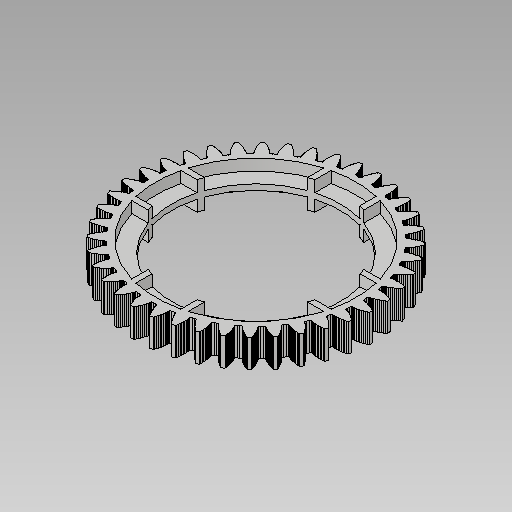
# Autodesk Inventor part: gear40
Saved by Autodesk Inventor 2020 (Build 240168000, 168)
## iProperties
Created: 2018-12-28
Part Number: gear40
Material: Generic
Document SubType Name: Modeling
Designer: Varga Daniel
Density: 1 g/cm^3
Appearance: Default
Sending System: SolidWorks 2018
Last Author: david
Last Saved: 2018-12-28
Author: Varga Daniel
Autodesk Inventor part; units mm, degrees
(part 1 of 3)
ref_plane "YZ Plane" through (0, 0, 0) normal (1, 0, 0) x (0, 1, 0)
ref_plane "XZ Plane" through (0, 0, 0) normal (0, 1, 0) x (-1, 0, 0)
ref_plane "XY Plane" through (0, 0, 0) normal (0, 0, 1) x (1, 0, 0)
sketch "Gear 40 tooth shape" plane through (0, 0, 0) normal (0, 0, 1) x (1, 0, 0)
  line L0 (2.4506, 21.4015) -> (2.3942, 21.6857)
  line L1 (2.3942, 21.6857) -> (2.3331, 21.6926)
  line L2 (2.3331, 21.6926) -> (2.2721, 21.7014)
  line L3 (2.2721, 21.7014) -> (2.1501, 21.7236)
  line L4 (2.1501, 21.7236) -> (2.0283, 21.7505)
  line L5 (2.0283, 21.7505) -> (1.9066, 21.7815)
  line L6 (1.9066, 21.7815) -> (1.6637, 21.8541)
  line L7 (1.6637, 21.8541) -> (1.4215, 21.9391)
  line L8 (1.4215, 21.9391) -> (1.18, 22.0351)
  line L9 (1.18, 22.0351) -> (0.9394, 22.1414)
  line L10 (0.9394, 22.1414) -> (0.6996, 22.2573)
  line L11 (0.6996, 22.2573) -> (0.461, 22.3824)
  line L12 (0.461, 22.3824) -> (0.2234, 22.5162)
  line L13 (0.2234, 22.5162) -> (0.046, 22.6222)
  line L14 (0.046, 22.6222) -> (0.0882, 23.1579)
  line L15 (0.0882, 23.1579) -> (0.2799, 23.2348)
  line L16 (0.2799, 23.2348) -> (0.5355, 23.3299)
  line L17 (0.5355, 23.3299) -> (0.7908, 23.4161)
  line L18 (0.7908, 23.4161) -> (1.0457, 23.4931)
  line L19 (1.0457, 23.4931) -> (1.3001, 23.5604)
  line L20 (1.3001, 23.5604) -> (1.5536, 23.6175)
  line L21 (1.5536, 23.6175) -> (1.8061, 23.6635)
  line L22 (1.8061, 23.6635) -> (2.0574, 23.6972)
  line L23 (2.0574, 23.6972) -> (2.1824, 23.7088)
  line L24 (2.1824, 23.7088) -> (2.3069, 23.7163)
  line L25 (2.3069, 23.7163) -> (2.4309, 23.7191)
  line L26 (2.4309, 23.7191) -> (2.4925, 23.7183)
  line L27 (2.4925, 23.7183) -> (2.554, 23.7155)
  line L28 (2.554, 23.7155) -> (2.6542, 23.9874)
  line L29 (2.6542, 23.9874) -> (2.7094, 24.3363)
  line L30 (2.7094, 24.3363) -> (2.6981, 24.6258)
  line L31 (2.6981, 24.6258) -> (2.6389, 24.6422)
  line L32 (2.6389, 24.6422) -> (2.58, 24.6605)
  line L33 (2.58, 24.6605) -> (2.463, 24.7014)
  line L34 (2.463, 24.7014) -> (2.3469, 24.7471)
  line L35 (2.3469, 24.7471) -> (2.2315, 24.7967)
  line L36 (2.2315, 24.7967) -> (2.003, 24.9064)
  line L37 (2.003, 24.9064) -> (1.777, 25.0282)
  line L38 (1.777, 25.0282) -> (1.5536, 25.1608)
  line L39 (1.5536, 25.1608) -> (1.3325, 25.3035)
  line L40 (1.3325, 25.3035) -> (1.1139, 25.4555)
  line L41 (1.1139, 25.4555) -> (0.8977, 25.6163)
  line L42 (0.8977, 25.6163) -> (0.684, 25.7857)
  line L43 (0.684, 25.7857) -> (0.5254, 25.9181)
  line L44 (0.5254, 25.9181) -> (0.6508, 26.4406)
  line L45 (0.6508, 26.4406) -> (0.8522, 26.4866)
  line L46 (0.8522, 26.4866) -> (1.1195, 26.5405)
  line L47 (1.1195, 26.5405) -> (1.3852, 26.5857)
  line L48 (1.3852, 26.5857) -> (1.649, 26.6219)
  line L49 (1.649, 26.6219) -> (1.9107, 26.6486)
  line L50 (1.9107, 26.6486) -> (2.1701, 26.6653)
  line L51 (2.1701, 26.6653) -> (2.4267, 26.6713)
  line L52 (2.4267, 26.6713) -> (2.6801, 26.6652)
  line L53 (2.6801, 26.6652) -> (2.8054, 26.6571)
  line L54 (2.8054, 26.6571) -> (2.9296, 26.6451)
  line L55 (2.9296, 26.6451) -> (3.0524, 26.6284)
  line L56 (3.0524, 26.6284) -> (3.1132, 26.618)
  line L57 (3.1132, 26.618) -> (3.1734, 26.6057)
  line L58 (3.1734, 26.6057) -> (3.315, 26.8585)
  line L59 (3.315, 26.8585) -> (3.4241, 27.1944)
  line L60 (3.4241, 27.1944) -> (3.4583, 27.4822)
  line L61 (3.4583, 27.4822) -> (3.4023, 27.5076)
  line L62 (3.4023, 27.5076) -> (3.3469, 27.5349)
  line L63 (3.3469, 27.5349) -> (3.2378, 27.5936)
  line L64 (3.2378, 27.5936) -> (3.1303, 27.6569)
  line L65 (3.1303, 27.6569) -> (3.0241, 27.724)
  line L66 (3.0241, 27.724) -> (2.8156, 27.868)
  line L67 (2.8156, 27.868) -> (2.6115, 28.0237)
  line L68 (2.6115, 28.0237) -> (2.4115, 28.1897)
  line L69 (2.4115, 28.1897) -> (2.2154, 28.3651)
  line L70 (2.2154, 28.3651) -> (2.0233, 28.5494)
  line L71 (2.0233, 28.5494) -> (1.8349, 28.7421)
  line L72 (1.8349, 28.7421) -> (1.6503, 28.9428)
  line L73 (1.6503, 28.9428) -> (1.5144, 29.0984)
  line L74 (1.5144, 29.0984) -> (1.72, 29.5949)
  line L75 (1.72, 29.5949) -> (1.9262, 29.6088)
  line L76 (1.9262, 29.6088) -> (2.1986, 29.6202)
  line L77 (2.1986, 29.6202) -> (2.4681, 29.6233)
  line L78 (2.4681, 29.6233) -> (2.7343, 29.6178)
  line L79 (2.7343, 29.6178) -> (2.997, 29.6032)
  line L80 (2.997, 29.6032) -> (3.2557, 29.5791)
  line L81 (3.2557, 29.5791) -> (3.5101, 29.5449)
  line L82 (3.5101, 29.5449) -> (3.7595, 29.4993)
  line L83 (3.7595, 29.4993) -> (3.882, 29.4717)
  line L84 (3.882, 29.4717) -> (4.0027, 29.4404)
  line L85 (4.0027, 29.4404) -> (4.1215, 29.4047)
  line L86 (4.1215, 29.4047) -> (4.1799, 29.3849)
  line L87 (4.1799, 29.3849) -> (4.2374, 29.3633)
  line L88 (4.2374, 29.3633) -> (4.4167, 29.5909)
  line L89 (4.4167, 29.5909) -> (4.5771, 29.9056)
  line L90 (4.5771, 29.9056) -> (4.6558, 30.1845)
  line L91 (4.6558, 30.1845) -> (4.6045, 30.2183)
  line L92 (4.6045, 30.2183) -> (4.5541, 30.2539)
  line L93 (4.5541, 30.2539) -> (4.4555, 30.329)
  line L94 (4.4555, 30.329) -> (4.3592, 30.4083)
  line L95 (4.3592, 30.4083) -> (4.2649, 30.4912)
  line L96 (4.2649, 30.4912) -> (4.0814, 30.6661)
  line L97 (4.0814, 30.6661) -> (3.9042, 30.8518)
  line L98 (3.9042, 30.8518) -> (3.7326, 31.047)
  line L99 (3.7326, 31.047) -> (3.5664, 31.2509)
  line L100 (3.5664, 31.2509) -> (3.4055, 31.4631)
  line L101 (3.4055, 31.4631) -> (3.2496, 31.6829)
  line L102 (3.2496, 31.6829) -> (3.0987, 31.91)
  line L103 (3.0987, 31.91) -> (2.9888, 32.0849)
  line L104 (2.9888, 32.0849) -> (3.2695, 32.5431)
  line L105 (3.2695, 32.5431) -> (3.4753, 32.5246)
  line L106 (3.4753, 32.5246) -> (3.7462, 32.4932)
  line L107 (3.7462, 32.4932) -> (4.0128, 32.4541)
  line L108 (4.0128, 32.4541) -> (4.2749, 32.407)
  line L109 (4.2749, 32.407) -> (4.532, 32.3515)
  line L110 (4.532, 32.3515) -> (4.7839, 32.2873)
  line L111 (4.7839, 32.2873) -> (5.0298, 32.2137)
  line L112 (5.0298, 32.2137) -> (5.2689, 32.1296)
  line L113 (5.2689, 32.1296) -> (5.3856, 32.0832)
  line L114 (5.3856, 32.0832) -> (5.5, 32.0334)
  line L115 (5.5, 32.0334) -> (5.6116, 31.9796)
  line L116 (5.6116, 31.9796) -> (5.6662, 31.9509)
  line L117 (5.6662, 31.9509) -> (5.7197, 31.9205)
  line L118 (5.7197, 31.9205) -> (5.9324, 32.1173)
  line L119 (5.9324, 32.1173) -> (6.14, 32.403)
  line L120 (6.14, 32.403) -> (6.2614, 32.6661)
  line L121 (6.2614, 32.6661) -> (6.216, 32.7076)
  line L122 (6.216, 32.7076) -> (6.1718, 32.7506)
  line L123 (6.1718, 32.7506) -> (6.0862, 32.8402)
  line L124 (6.0862, 32.8402) -> (6.0035, 32.9336)
  line L125 (6.0035, 32.9336) -> (5.9233, 33.0302)
  line L126 (5.9233, 33.0302) -> (5.7694, 33.2317)
  line L127 (5.7694, 33.2317) -> (5.6234, 33.4428)
  line L128 (5.6234, 33.4428) -> (5.4845, 33.6624)
  line L129 (5.4845, 33.6624) -> (5.3523, 33.8899)
  line L130 (5.3523, 33.8899) -> (5.2265, 34.1246)
  line L131 (5.2265, 34.1246) -> (5.1069, 34.3661)
  line L132 (5.1069, 34.3661) -> (4.9934, 34.614)
  line L133 (4.9934, 34.614) -> (4.9122, 34.804)
  line L134 (4.9122, 34.804) -> (5.2611, 35.2126)
  line L135 (5.2611, 35.2126) -> (5.4615, 35.1621)
  line L136 (5.4615, 35.1621) -> (5.7241, 35.0888)
  line L137 (5.7241, 35.0888) -> (5.9813, 35.0084)
  line L138 (5.9813, 35.0084) -> (6.2328, 34.9209)
  line L139 (6.2328, 34.9209) -> (6.4781, 34.8259)
  line L140 (6.4781, 34.8259) -> (6.7168, 34.723)
  line L141 (6.7168, 34.723) -> (6.9482, 34.6118)
  line L142 (6.9482, 34.6118) -> (7.1712, 34.4914)
  line L143 (7.1712, 34.4914) -> (7.2792, 34.4273)
  line L144 (7.2792, 34.4273) -> (7.3844, 34.3602)
  line L145 (7.3844, 34.3602) -> (7.4863, 34.2896)
  line L146 (7.4863, 34.2896) -> (7.5357, 34.2527)
  line L147 (7.5357, 34.2527) -> (7.5837, 34.2144)
  line L148 (7.5837, 34.2144) -> (7.8246, 34.3754)
  line L149 (7.8246, 34.3754) -> (8.0744, 34.6252)
  line L150 (8.0744, 34.6252) -> (8.2354, 34.8661)
  line L151 (8.2354, 34.8661) -> (8.1971, 34.9141)
  line L152 (8.1971, 34.9141) -> (8.1602, 34.9635)
  line L153 (8.1602, 34.9635) -> (8.0896, 35.0654)
  line L154 (8.0896, 35.0654) -> (8.0225, 35.1706)
  line L155 (8.0225, 35.1706) -> (7.9584, 35.2786)
  line L156 (7.9584, 35.2786) -> (7.838, 35.5016)
  line L157 (7.838, 35.5016) -> (7.7268, 35.733)
  line L158 (7.7268, 35.733) -> (7.6239, 35.9717)
  line L159 (7.6239, 35.9717) -> (7.5289, 36.217)
  line L160 (7.5289, 36.217) -> (7.4414, 36.4685)
  line L161 (7.4414, 36.4685) -> (7.361, 36.7257)
  line L162 (7.361, 36.7257) -> (7.2877, 36.9883)
  line L163 (7.2877, 36.9883) -> (7.2372, 37.1887)
  line L164 (7.2372, 37.1887) -> (7.6459, 37.5377)
  line L165 (7.6459, 37.5377) -> (7.8358, 37.4565)
  line L166 (7.8358, 37.4565) -> (8.0837, 37.343)
  line L167 (8.0837, 37.343) -> (8.3252, 37.2234)
  line L168 (8.3252, 37.2234) -> (8.5599, 37.0975)
  line L169 (8.5599, 37.0975) -> (8.7874, 36.9653)
  line L170 (8.7874, 36.9653) -> (9.007, 36.8264)
  line L171 (9.007, 36.8264) -> (9.2181, 36.6804)
  line L172 (9.2181, 36.6804) -> (9.4196, 36.5266)
  line L173 (9.4196, 36.5266) -> (9.5162, 36.4464)
  line L174 (9.5162, 36.4464) -> (9.6096, 36.3636)
  line L175 (9.6096, 36.3636) -> (9.6992, 36.278)
  line L176 (9.6992, 36.278) -> (9.7422, 36.2338)
  line L177 (9.7422, 36.2338) -> (9.7837, 36.1884)
  line L178 (9.7837, 36.1884) -> (10.0468, 36.3098)
  line L179 (10.0468, 36.3098) -> (10.3326, 36.5174)
  line L180 (10.3326, 36.5174) -> (10.5293, 36.7301)
  line L181 (10.5293, 36.7301) -> (10.499, 36.7836)
  line L182 (10.499, 36.7836) -> (10.4702, 36.8382)
  line L183 (10.4702, 36.8382) -> (10.4164, 36.9499)
  line L184 (10.4164, 36.9499) -> (10.3666, 37.0642)
  line L185 (10.3666, 37.0642) -> (10.3202, 37.1809)
  line L186 (10.3202, 37.1809) -> (10.2362, 37.4201)
  line L187 (10.2362, 37.4201) -> (10.1625, 37.666)
  line L188 (10.1625, 37.666) -> (10.0983, 37.9178)
  line L189 (10.0983, 37.9178) -> (10.0428, 38.175)
  line L190 (10.0428, 38.175) -> (9.9957, 38.437)
  line L191 (9.9957, 38.437) -> (9.9566, 38.7037)
  line L192 (9.9566, 38.7037) -> (9.9252, 38.9745)
  line L193 (9.9252, 38.9745) -> (9.9067, 39.1803)
  line L194 (9.9067, 39.1803) -> (10.3649, 39.4611)
  line L195 (10.3649, 39.4611) -> (10.5398, 39.3511)
  line L196 (10.5398, 39.3511) -> (10.7669, 39.2002)
  line L197 (10.7669, 39.2002) -> (10.9868, 39.0443)
  line L198 (10.9868, 39.0443) -> (11.1989, 38.8834)
  line L199 (11.1989, 38.8834) -> (11.4028, 38.7172)
  line L200 (11.4028, 38.7172) -> (11.5981, 38.5456)
  line L201 (11.5981, 38.5456) -> (11.7837, 38.3684)
  line L202 (11.7837, 38.3684) -> (11.9586, 38.1849)
  line L203 (11.9586, 38.1849) -> (12.0415, 38.0906)
  line L204 (12.0415, 38.0906) -> (12.1208, 37.9943)
  line L205 (12.1208, 37.9943) -> (12.1959, 37.8957)
  line L206 (12.1959, 37.8957) -> (12.2315, 37.8453)
  line L207 (12.2315, 37.8453) -> (12.2654, 37.794)
  line L208 (12.2654, 37.794) -> (12.5442, 37.8727)
  line L209 (12.5442, 37.8727) -> (12.8589, 38.0331)
  line L210 (12.8589, 38.0331) -> (13.0865, 38.2124)
  line L211 (13.0865, 38.2124) -> (13.0649, 38.27)
  line L212 (13.0649, 38.27) -> (13.0451, 38.3284)
  line L213 (13.0451, 38.3284) -> (13.0095, 38.4471)
  line L214 (13.0095, 38.4471) -> (12.9781, 38.5678)
  line L215 (12.9781, 38.5678) -> (12.9505, 38.6903)
  line L216 (12.9505, 38.6903) -> (12.9049, 38.9397)
  line L217 (12.9049, 38.9397) -> (12.8707, 39.1941)
  line L218 (12.8707, 39.1941) -> (12.8466, 39.4528)
  line L219 (12.8466, 39.4528) -> (12.8321, 39.7155)
  line L220 (12.8321, 39.7155) -> (12.8265, 39.9817)
  line L221 (12.8265, 39.9817) -> (12.8296, 40.2512)
  line L222 (12.8296, 40.2512) -> (12.841, 40.5236)
  line L223 (12.841, 40.5236) -> (12.8549, 40.7298)
  line L224 (12.8549, 40.7298) -> (13.3514, 40.9354)
  line L225 (13.3514, 40.9354) -> (13.507, 40.7995)
  line L226 (13.507, 40.7995) -> (13.7077, 40.6149)
  line L227 (13.7077, 40.6149) -> (13.9004, 40.4266)
  line L228 (13.9004, 40.4266) -> (14.0847, 40.2344)
  line L229 (14.0847, 40.2344) -> (14.2601, 40.0384)
  line L230 (14.2601, 40.0384) -> (14.4261, 39.8384)
  line L231 (14.4261, 39.8384) -> (14.5818, 39.6343)
  line L232 (14.5818, 39.6343) -> (14.7259, 39.4257)
  line L233 (14.7259, 39.4257) -> (14.7929, 39.3196)
  line L234 (14.7929, 39.3196) -> (14.8562, 39.212)
  line L235 (14.8562, 39.212) -> (14.915, 39.1029)
  line L236 (14.915, 39.1029) -> (14.9422, 39.0476)
  line L237 (14.9422, 39.0476) -> (14.9676, 38.9916)
  line L238 (14.9676, 38.9916) -> (15.2554, 39.0257)
  line L239 (15.2554, 39.0257) -> (15.5913, 39.1349)
  line L240 (15.5913, 39.1349) -> (15.8442, 39.2764)
  line L241 (15.8442, 39.2764) -> (15.8318, 39.3366)
  line L242 (15.8318, 39.3366) -> (15.8214, 39.3974)
  line L243 (15.8214, 39.3974) -> (15.8047, 39.5202)
  line L244 (15.8047, 39.5202) -> (15.7927, 39.6444)
  line L245 (15.7927, 39.6444) -> (15.7846, 39.7697)
  line L246 (15.7846, 39.7697) -> (15.7786, 40.0231)
  line L247 (15.7786, 40.0231) -> (15.7845, 40.2797)
  line L248 (15.7845, 40.2797) -> (15.8012, 40.5391)
  line L249 (15.8012, 40.5391) -> (15.828, 40.8008)
  line L250 (15.828, 40.8008) -> (15.8641, 41.0646)
  line L251 (15.8641, 41.0646) -> (15.9093, 41.3303)
  line L252 (15.9093, 41.3303) -> (15.9632, 41.5976)
  line L253 (15.9632, 41.5976) -> (16.0092, 41.799)
  line L254 (16.0092, 41.799) -> (16.5317, 41.9244)
  line L255 (16.5317, 41.9244) -> (16.6641, 41.7658)
  line L256 (16.6641, 41.7658) -> (16.8335, 41.5521)
  line L257 (16.8335, 41.5521) -> (16.9944, 41.336)
  line L258 (16.9944, 41.336) -> (17.1463, 41.1173)
  line L259 (17.1463, 41.1173) -> (17.289, 40.8963)
  line L260 (17.289, 40.8963) -> (17.4216, 40.6728)
  line L261 (17.4216, 40.6728) -> (17.5434, 40.4468)
  line L262 (17.5434, 40.4468) -> (17.6531, 40.2183)
  line L263 (17.6531, 40.2183) -> (17.7028, 40.103)
  line L264 (17.7028, 40.103) -> (17.7484, 39.9869)
  line L265 (17.7484, 39.9869) -> (17.7894, 39.8699)
  line L266 (17.7894, 39.8699) -> (17.8076, 39.8109)
  line L267 (17.8076, 39.8109) -> (17.824, 39.7517)
  line L268 (17.824, 39.7517) -> (18.1135, 39.7404)
  line L269 (18.1135, 39.7404) -> (18.4624, 39.7957)
  line L270 (18.4624, 39.7957) -> (18.7343, 39.8959)
  line L271 (18.7343, 39.8959) -> (18.7315, 39.9573)
  line L272 (18.7315, 39.9573) -> (18.7307, 40.019)
  line L273 (18.7307, 40.019) -> (18.7335, 40.1429)
  line L274 (18.7335, 40.1429) -> (18.741, 40.2674)
  line L275 (18.741, 40.2674) -> (18.7526, 40.3924)
  line L276 (18.7526, 40.3924) -> (18.7863, 40.6437)
  line L277 (18.7863, 40.6437) -> (18.8323, 40.8962)
  line L278 (18.8323, 40.8962) -> (18.8894, 41.1497)
  line L279 (18.8894, 41.1497) -> (18.9568, 41.4041)
  line L280 (18.9568, 41.4041) -> (19.0338, 41.659)
  line L281 (19.0338, 41.659) -> (19.1199, 41.9143)
  line L282 (19.1199, 41.9143) -> (19.215, 42.1699)
  line L283 (19.215, 42.1699) -> (19.2919, 42.3616)
  line L284 (19.2919, 42.3616) -> (19.8276, 42.4038)
  line L285 (19.8276, 42.4038) -> (19.9336, 42.2264)
  line L286 (19.9336, 42.2264) -> (20.0674, 41.9889)
  line L287 (20.0674, 41.9889) -> (20.1925, 41.7502)
  line L288 (20.1925, 41.7502) -> (20.3084, 41.5104)
  line L289 (20.3084, 41.5104) -> (20.4147, 41.2698)
  line L290 (20.4147, 41.2698) -> (20.5108, 41.0283)
  line L291 (20.5108, 41.0283) -> (20.5957, 40.7861)
  line L292 (20.5957, 40.7861) -> (20.6683, 40.5432)
  line L293 (20.6683, 40.5432) -> (20.6993, 40.4215)
  line L294 (20.6993, 40.4215) -> (20.7262, 40.2997)
  line L295 (20.7262, 40.2997) -> (20.7484, 40.1778)
  line L296 (20.7484, 40.1778) -> (20.7572, 40.1167)
  line L297 (20.7572, 40.1167) -> (20.7641, 40.0556)
  line L298 (20.7641, 40.0556) -> (21.0483, 39.9992)
  line L299 (21.0483, 39.9992) -> (21.4015, 39.9992)
  line L300 (21.4015, 39.9992) -> (21.6857, 40.0556)
  line L301 (21.6857, 40.0556) -> (21.6926, 40.1167)
  line L302 (21.6926, 40.1167) -> (21.7014, 40.1778)
  line L303 (21.7014, 40.1778) -> (21.7236, 40.2997)
  line L304 (21.7236, 40.2997) -> (21.7505, 40.4215)
  line L305 (21.7505, 40.4215) -> (21.7815, 40.5432)
  line L306 (21.7815, 40.5432) -> (21.8541, 40.7861)
  line L307 (21.8541, 40.7861) -> (21.9391, 41.0283)
  line L308 (21.9391, 41.0283) -> (22.0351, 41.2698)
  line L309 (22.0351, 41.2698) -> (22.1414, 41.5104)
  line L310 (22.1414, 41.5104) -> (22.2573, 41.7502)
  line L311 (22.2573, 41.7502) -> (22.3824, 41.9889)
  line L312 (22.3824, 41.9889) -> (22.5162, 42.2264)
  line L313 (22.5162, 42.2264) -> (22.6222, 42.4038)
  line L314 (22.6222, 42.4038) -> (23.1579, 42.3616)
  line L315 (23.1579, 42.3616) -> (23.2348, 42.1699)
  line L316 (23.2348, 42.1699) -> (23.3299, 41.9143)
  line L317 (23.3299, 41.9143) -> (23.4161, 41.659)
  line L318 (23.4161, 41.659) -> (23.4931, 41.4041)
  line L319 (23.4931, 41.4041) -> (23.5604, 41.1497)
  line L320 (23.5604, 41.1497) -> (23.6175, 40.8962)
  line L321 (23.6175, 40.8962) -> (23.6635, 40.6437)
  line L322 (23.6635, 40.6437) -> (23.6972, 40.3924)
  line L323 (23.6972, 40.3924) -> (23.7088, 40.2674)
  line L324 (23.7088, 40.2674) -> (23.7163, 40.1429)
  line L325 (23.7163, 40.1429) -> (23.7191, 40.019)
  line L326 (23.7191, 40.019) -> (23.7183, 39.9573)
  line L327 (23.7183, 39.9573) -> (23.7155, 39.8959)
  line L328 (23.7155, 39.8959) -> (23.9874, 39.7957)
  line L329 (23.9874, 39.7957) -> (24.3363, 39.7404)
  line L330 (24.3363, 39.7404) -> (24.6258, 39.7517)
  line L331 (24.6258, 39.7517) -> (24.6422, 39.8109)
  line L332 (24.6422, 39.8109) -> (24.6605, 39.8699)
  line L333 (24.6605, 39.8699) -> (24.7014, 39.9869)
  line L334 (24.7014, 39.9869) -> (24.7471, 40.103)
  line L335 (24.7471, 40.103) -> (24.7967, 40.2183)
  line L336 (24.7967, 40.2183) -> (24.9064, 40.4468)
  line L337 (24.9064, 40.4468) -> (25.0282, 40.6728)
  line L338 (25.0282, 40.6728) -> (25.1608, 40.8963)
  line L339 (25.1608, 40.8963) -> (25.3035, 41.1173)
  line L340 (25.3035, 41.1173) -> (25.4555, 41.336)
  line L341 (25.4555, 41.336) -> (25.6163, 41.5521)
  line L342 (25.6163, 41.5521) -> (25.7857, 41.7658)
  line L343 (25.7857, 41.7658) -> (25.9181, 41.9244)
  line L344 (25.9181, 41.9244) -> (26.4406, 41.799)
  line L345 (26.4406, 41.799) -> (26.4866, 41.5976)
  line L346 (26.4866, 41.5976) -> (26.5405, 41.3303)
  line L347 (26.5405, 41.3303) -> (26.5857, 41.0646)
  line L348 (26.5857, 41.0646) -> (26.6219, 40.8008)
  line L349 (26.6219, 40.8008) -> (26.6486, 40.5391)
  line L350 (26.6486, 40.5391) -> (26.6653, 40.2797)
  line L351 (26.6653, 40.2797) -> (26.6713, 40.0231)
  line L352 (26.6713, 40.0231) -> (26.6652, 39.7697)
  line L353 (26.6652, 39.7697) -> (26.6571, 39.6444)
  line L354 (26.6571, 39.6444) -> (26.6451, 39.5202)
  line L355 (26.6451, 39.5202) -> (26.6284, 39.3974)
  line L356 (26.6284, 39.3974) -> (26.618, 39.3366)
  line L357 (26.618, 39.3366) -> (26.6057, 39.2764)
  line L358 (26.6057, 39.2764) -> (26.8585, 39.1349)
  line L359 (26.8585, 39.1349) -> (27.1944, 39.0257)
  line L360 (27.1944, 39.0257) -> (27.4822, 38.9916)
  line L361 (27.4822, 38.9916) -> (27.5076, 39.0476)
  line L362 (27.5076, 39.0476) -> (27.5349, 39.1029)
  line L363 (27.5349, 39.1029) -> (27.5936, 39.212)
  line L364 (27.5936, 39.212) -> (27.6569, 39.3196)
  line L365 (27.6569, 39.3196) -> (27.724, 39.4257)
  line L366 (27.724, 39.4257) -> (27.868, 39.6343)
  line L367 (27.868, 39.6343) -> (28.0237, 39.8384)
  line L368 (28.0237, 39.8384) -> (28.1897, 40.0384)
  line L369 (28.1897, 40.0384) -> (28.3651, 40.2344)
  line L370 (28.3651, 40.2344) -> (28.5494, 40.4266)
  line L371 (28.5494, 40.4266) -> (28.7421, 40.6149)
  line L372 (28.7421, 40.6149) -> (28.9428, 40.7995)
  line L373 (28.9428, 40.7995) -> (29.0984, 40.9354)
  line L374 (29.0984, 40.9354) -> (29.5949, 40.7298)
  line L375 (29.5949, 40.7298) -> (29.6088, 40.5236)
  line L376 (29.6088, 40.5236) -> (29.6202, 40.2512)
  line L377 (29.6202, 40.2512) -> (29.6233, 39.9817)
  line L378 (29.6233, 39.9817) -> (29.6178, 39.7155)
  line L379 (29.6178, 39.7155) -> (29.6032, 39.4528)
  line L380 (29.6032, 39.4528) -> (29.5791, 39.1941)
  line L381 (29.5791, 39.1941) -> (29.5449, 38.9397)
  line L382 (29.5449, 38.9397) -> (29.4993, 38.6903)
  line L383 (29.4993, 38.6903) -> (29.4717, 38.5678)
  line L384 (29.4717, 38.5678) -> (29.4404, 38.4471)
  line L385 (29.4404, 38.4471) -> (29.4047, 38.3284)
  line L386 (29.4047, 38.3284) -> (29.3849, 38.27)
  line L387 (29.3849, 38.27) -> (29.3633, 38.2124)
  line L388 (29.3633, 38.2124) -> (29.5909, 38.0331)
  line L389 (29.5909, 38.0331) -> (29.9056, 37.8727)
  line L390 (29.9056, 37.8727) -> (30.1845, 37.794)
  line L391 (30.1845, 37.794) -> (30.2183, 37.8453)
  line L392 (30.2183, 37.8453) -> (30.2539, 37.8957)
  line L393 (30.2539, 37.8957) -> (30.329, 37.9943)
  line L394 (30.329, 37.9943) -> (30.4083, 38.0906)
  line L395 (30.4083, 38.0906) -> (30.4912, 38.1849)
  line L396 (30.4912, 38.1849) -> (30.6661, 38.3684)
  line L397 (30.6661, 38.3684) -> (30.8518, 38.5456)
  line L398 (30.8518, 38.5456) -> (31.047, 38.7172)
  line L399 (31.047, 38.7172) -> (31.2509, 38.8834)
  line L400 (31.2509, 38.8834) -> (31.4631, 39.0443)
  line L401 (31.4631, 39.0443) -> (31.6829, 39.2002)
  line L402 (31.6829, 39.2002) -> (31.91, 39.3511)
  line L403 (31.91, 39.3511) -> (32.0849, 39.4611)
  line L404 (32.0849, 39.4611) -> (32.5431, 39.1803)
  line L405 (32.5431, 39.1803) -> (32.5246, 38.9745)
  line L406 (32.5246, 38.9745) -> (32.4932, 38.7037)
  line L407 (32.4932, 38.7037) -> (32.4541, 38.437)
  line L408 (32.4541, 38.437) -> (32.407, 38.175)
  line L409 (32.407, 38.175) -> (32.3515, 37.9178)
  line L410 (32.3515, 37.9178) -> (32.2873, 37.666)
  line L411 (32.2873, 37.666) -> (32.2137, 37.4201)
  line L412 (32.2137, 37.4201) -> (32.1296, 37.1809)
  line L413 (32.1296, 37.1809) -> (32.0832, 37.0642)
  line L414 (32.0832, 37.0642) -> (32.0334, 36.9499)
  line L415 (32.0334, 36.9499) -> (31.9796, 36.8382)
  line L416 (31.9796, 36.8382) -> (31.9509, 36.7836)
  line L417 (31.9509, 36.7836) -> (31.9205, 36.7301)
  line L418 (31.9205, 36.7301) -> (32.1173, 36.5174)
  line L419 (32.1173, 36.5174) -> (32.403, 36.3098)
  line L420 (32.403, 36.3098) -> (32.6661, 36.1884)
  line L421 (32.6661, 36.1884) -> (32.7076, 36.2338)
  line L422 (32.7076, 36.2338) -> (32.7506, 36.278)
  line L423 (32.7506, 36.278) -> (32.8402, 36.3636)
  line L424 (32.8402, 36.3636) -> (32.9336, 36.4464)
  line L425 (32.9336, 36.4464) -> (33.0302, 36.5266)
  line L426 (33.0302, 36.5266) -> (33.2317, 36.6804)
  line L427 (33.2317, 36.6804) -> (33.4428, 36.8264)
  line L428 (33.4428, 36.8264) -> (33.6624, 36.9653)
  line L429 (33.6624, 36.9653) -> (33.8899, 37.0975)
  line L430 (33.8899, 37.0975) -> (34.1246, 37.2234)
  line L431 (34.1246, 37.2234) -> (34.3661, 37.343)
  line L432 (34.3661, 37.343) -> (34.614, 37.4565)
  line L433 (34.614, 37.4565) -> (34.804, 37.5377)
  line L434 (34.804, 37.5377) -> (35.2126, 37.1887)
  line L435 (35.2126, 37.1887) -> (35.1621, 36.9883)
  line L436 (35.1621, 36.9883) -> (35.0888, 36.7257)
  line L437 (35.0888, 36.7257) -> (35.0084, 36.4685)
  line L438 (35.0084, 36.4685) -> (34.9209, 36.217)
  line L439 (34.9209, 36.217) -> (34.8259, 35.9717)
  line L440 (34.8259, 35.9717) -> (34.723, 35.733)
  line L441 (34.723, 35.733) -> (34.6118, 35.5016)
  line L442 (34.6118, 35.5016) -> (34.4914, 35.2786)
  line L443 (34.4914, 35.2786) -> (34.4273, 35.1706)
  line L444 (34.4273, 35.1706) -> (34.3602, 35.0654)
  line L445 (34.3602, 35.0654) -> (34.2896, 34.9635)
  line L446 (34.2896, 34.9635) -> (34.2527, 34.9141)
  line L447 (34.2527, 34.9141) -> (34.2144, 34.8661)
  line L448 (34.2144, 34.8661) -> (34.3754, 34.6252)
  line L449 (34.3754, 34.6252) -> (34.6252, 34.3754)
  line L450 (34.6252, 34.3754) -> (34.8661, 34.2144)
  line L451 (34.8661, 34.2144) -> (34.9141, 34.2527)
  line L452 (34.9141, 34.2527) -> (34.9635, 34.2896)
  line L453 (34.9635, 34.2896) -> (35.0654, 34.3602)
  line L454 (35.0654, 34.3602) -> (35.1706, 34.4273)
  line L455 (35.1706, 34.4273) -> (35.2786, 34.4914)
  line L456 (35.2786, 34.4914) -> (35.5016, 34.6118)
  line L457 (35.5016, 34.6118) -> (35.733, 34.723)
  line L458 (35.733, 34.723) -> (35.9717, 34.8259)
  line L459 (35.9717, 34.8259) -> (36.217, 34.9209)
  line L460 (36.217, 34.9209) -> (36.4685, 35.0084)
  line L461 (36.4685, 35.0084) -> (36.7257, 35.0888)
  line L462 (36.7257, 35.0888) -> (36.9883, 35.1621)
  line L463 (36.9883, 35.1621) -> (37.1887, 35.2126)
  line L464 (37.1887, 35.2126) -> (37.5377, 34.804)
  line L465 (37.5377, 34.804) -> (37.4565, 34.614)
  line L466 (37.4565, 34.614) -> (37.343, 34.3661)
  line L467 (37.343, 34.3661) -> (37.2234, 34.1246)
  line L468 (37.2234, 34.1246) -> (37.0975, 33.8899)
  line L469 (37.0975, 33.8899) -> (36.9653, 33.6624)
  line L470 (36.9653, 33.6624) -> (36.8264, 33.4428)
  line L471 (36.8264, 33.4428) -> (36.6804, 33.2317)
  line L472 (36.6804, 33.2317) -> (36.5266, 33.0302)
  line L473 (36.5266, 33.0302) -> (36.4464, 32.9336)
  line L474 (36.4464, 32.9336) -> (36.3636, 32.8402)
  line L475 (36.3636, 32.8402) -> (36.278, 32.7506)
  line L476 (36.278, 32.7506) -> (36.2338, 32.7076)
  line L477 (36.2338, 32.7076) -> (36.1884, 32.6661)
  line L478 (36.1884, 32.6661) -> (36.3098, 32.403)
  line L479 (36.3098, 32.403) -> (36.5174, 32.1173)
  line L480 (36.5174, 32.1173) -> (36.7301, 31.9205)
  line L481 (36.7301, 31.9205) -> (36.7836, 31.9509)
  line L482 (36.7836, 31.9509) -> (36.8382, 31.9796)
  line L483 (36.8382, 31.9796) -> (36.9499, 32.0334)
  line L484 (36.9499, 32.0334) -> (37.0642, 32.0832)
  line L485 (37.0642, 32.0832) -> (37.1809, 32.1296)
  line L486 (37.1809, 32.1296) -> (37.4201, 32.2137)
  line L487 (37.4201, 32.2137) -> (37.666, 32.2873)
  line L488 (37.666, 32.2873) -> (37.9178, 32.3515)
  line L489 (37.9178, 32.3515) -> (38.175, 32.407)
  line L490 (38.175, 32.407) -> (38.437, 32.4541)
  line L491 (38.437, 32.4541) -> (38.7037, 32.4932)
  line L492 (38.7037, 32.4932) -> (38.9745, 32.5246)
  line L493 (38.9745, 32.5246) -> (39.1803, 32.5431)
  line L494 (39.1803, 32.5431) -> (39.4611, 32.0849)
  line L495 (39.4611, 32.0849) -> (39.3511, 31.91)
  line L496 (39.3511, 31.91) -> (39.2002, 31.6829)
  line L497 (39.2002, 31.6829) -> (39.0443, 31.4631)
  line L498 (39.0443, 31.4631) -> (38.8834, 31.2509)
  line L499 (38.8834, 31.2509) -> (38.7172, 31.047)
  line L500 (38.7172, 31.047) -> (38.5456, 30.8518)
  line L501 (38.5456, 30.8518) -> (38.3684, 30.6661)
  line L502 (38.3684, 30.6661) -> (38.1849, 30.4912)
  line L503 (38.1849, 30.4912) -> (38.0906, 30.4083)
  line L504 (38.0906, 30.4083) -> (37.9943, 30.329)
  line L505 (37.9943, 30.329) -> (37.8957, 30.2539)
  line L506 (37.8957, 30.2539) -> (37.8453, 30.2183)
  line L507 (37.8453, 30.2183) -> (37.794, 30.1845)
  line L508 (37.794, 30.1845) -> (37.8727, 29.9056)
  line L509 (37.8727, 29.9056) -> (38.0331, 29.5909)
  line L510 (38.0331, 29.5909) -> (38.2124, 29.3633)
  line L511 (38.2124, 29.3633) -> (38.27, 29.3849)
  line L512 (38.27, 29.3849) -> (38.3284, 29.4047)
  line L513 (38.3284, 29.4047) -> (38.4471, 29.4404)
  line L514 (38.4471, 29.4404) -> (38.5678, 29.4717)
  line L515 (38.5678, 29.4717) -> (38.6903, 29.4993)
  line L516 (38.6903, 29.4993) -> (38.9397, 29.5449)
  line L517 (38.9397, 29.5449) -> (39.1941, 29.5791)
  line L518 (39.1941, 29.5791) -> (39.4528, 29.6032)
  line L519 (39.4528, 29.6032) -> (39.7155, 29.6178)
  line L520 (39.7155, 29.6178) -> (39.9817, 29.6233)
  line L521 (39.9817, 29.6233) -> (40.2512, 29.6202)
  line L522 (40.2512, 29.6202) -> (40.5236, 29.6088)
  line L523 (40.5236, 29.6088) -> (40.7298, 29.5949)
  line L524 (40.7298, 29.5949) -> (40.9354, 29.0984)
  line L525 (40.9354, 29.0984) -> (40.7995, 28.9428)
  line L526 (40.7995, 28.9428) -> (40.6149, 28.7421)
  line L527 (40.6149, 28.7421) -> (40.4266, 28.5494)
  line L528 (40.4266, 28.5494) -> (40.2344, 28.3651)
  line L529 (40.2344, 28.3651) -> (40.0384, 28.1897)
  line L530 (40.0384, 28.1897) -> (39.8384, 28.0237)
  line L531 (39.8384, 28.0237) -> (39.6343, 27.868)
  line L532 (39.6343, 27.868) -> (39.4257, 27.724)
  line L533 (39.4257, 27.724) -> (39.3196, 27.6569)
  line L534 (39.3196, 27.6569) -> (39.212, 27.5936)
  line L535 (39.212, 27.5936) -> (39.1029, 27.5349)
  line L536 (39.1029, 27.5349) -> (39.0476, 27.5076)
  line L537 (39.0476, 27.5076) -> (38.9916, 27.4822)
  line L538 (38.9916, 27.4822) -> (39.0257, 27.1944)
  line L539 (39.0257, 27.1944) -> (39.1349, 26.8585)
  line L540 (39.1349, 26.8585) -> (39.2764, 26.6057)
  line L541 (39.2764, 26.6057) -> (39.3366, 26.618)
  line L542 (39.3366, 26.618) -> (39.3974, 26.6284)
  line L543 (39.3974, 26.6284) -> (39.5202, 26.6451)
  line L544 (39.5202, 26.6451) -> (39.6444, 26.6571)
  line L545 (39.6444, 26.6571) -> (39.7697, 26.6652)
  line L546 (39.7697, 26.6652) -> (40.0231, 26.6713)
  line L547 (40.0231, 26.6713) -> (40.2797, 26.6653)
  line L548 (40.2797, 26.6653) -> (40.5391, 26.6486)
  line L549 (40.5391, 26.6486) -> (40.8008, 26.6219)
  line L550 (40.8008, 26.6219) -> (41.0646, 26.5857)
  line L551 (41.0646, 26.5857) -> (41.3303, 26.5405)
  line L552 (41.3303, 26.5405) -> (41.5976, 26.4866)
  line L553 (41.5976, 26.4866) -> (41.799, 26.4406)
  line L554 (41.799, 26.4406) -> (41.9244, 25.9181)
  line L555 (41.9244, 25.9181) -> (41.7658, 25.7857)
  line L556 (41.7658, 25.7857) -> (41.5521, 25.6163)
  line L557 (41.5521, 25.6163) -> (41.336, 25.4555)
  line L558 (41.336, 25.4555) -> (41.1173, 25.3035)
  line L559 (41.1173, 25.3035) -> (40.8963, 25.1608)
  line L560 (40.8963, 25.1608) -> (40.6728, 25.0282)
  line L561 (40.6728, 25.0282) -> (40.4468, 24.9064)
  line L562 (40.4468, 24.9064) -> (40.2183, 24.7967)
  line L563 (40.2183, 24.7967) -> (40.103, 24.7471)
  line L564 (40.103, 24.7471) -> (39.9869, 24.7014)
  line L565 (39.9869, 24.7014) -> (39.8699, 24.6605)
  line L566 (39.8699, 24.6605) -> (39.8109, 24.6422)
  line L567 (39.8109, 24.6422) -> (39.7517, 24.6258)
  line L568 (39.7517, 24.6258) -> (39.7404, 24.3363)
  line L569 (39.7404, 24.3363) -> (39.7957, 23.9874)
  line L570 (39.7957, 23.9874) -> (39.8959, 23.7155)
  line L571 (39.8959, 23.7155) -> (39.9573, 23.7183)
  line L572 (39.9573, 23.7183) -> (40.019, 23.7191)
  line L573 (40.019, 23.7191) -> (40.1429, 23.7163)
  line L574 (40.1429, 23.7163) -> (40.2674, 23.7088)
  line L575 (40.2674, 23.7088) -> (40.3924, 23.6972)
  line L576 (40.3924, 23.6972) -> (40.6437, 23.6635)
  line L577 (40.6437, 23.6635) -> (40.8962, 23.6175)
  line L578 (40.8962, 23.6175) -> (41.1497, 23.5604)
  line L579 (41.1497, 23.5604) -> (41.4041, 23.4931)
  line L580 (41.4041, 23.4931) -> (41.659, 23.4161)
  line L581 (41.659, 23.4161) -> (41.9143, 23.3299)
  line L582 (41.9143, 23.3299) -> (42.1699, 23.2348)
  line L583 (42.1699, 23.2348) -> (42.3616, 23.1579)
  line L584 (42.3616, 23.1579) -> (42.4038, 22.6222)
  line L585 (42.4038, 22.6222) -> (42.2264, 22.5162)
  line L586 (42.2264, 22.5162) -> (41.9889, 22.3824)
  line L587 (41.9889, 22.3824) -> (41.7502, 22.2573)
  line L588 (41.7502, 22.2573) -> (41.5104, 22.1414)
  line L589 (41.5104, 22.1414) -> (41.2698, 22.0351)
  line L590 (41.2698, 22.0351) -> (41.0283, 21.9391)
  line L591 (41.0283, 21.9391) -> (40.7861, 21.8541)
  line L592 (40.7861, 21.8541) -> (40.5432, 21.7815)
  line L593 (40.5432, 21.7815) -> (40.4215, 21.7505)
  line L594 (40.4215, 21.7505) -> (40.2997, 21.7236)
  line L595 (40.2997, 21.7236) -> (40.1778, 21.7014)
  line L596 (40.1778, 21.7014) -> (40.1167, 21.6926)
  line L597 (40.1167, 21.6926) -> (40.0556, 21.6857)
  line L598 (40.0556, 21.6857) -> (39.9992, 21.4015)
  line L599 (39.9992, 21.4015) -> (39.9992, 21.0483)
  line L600 (39.9992, 21.0483) -> (40.0556, 20.7641)
  line L601 (40.0556, 20.7641) -> (40.1167, 20.7572)
  line L602 (40.1167, 20.7572) -> (40.1778, 20.7484)
  line L603 (40.1778, 20.7484) -> (40.2997, 20.7262)
  line L604 (40.2997, 20.7262) -> (40.4215, 20.6993)
  line L605 (40.4215, 20.6993) -> (40.5432, 20.6683)
  line L606 (40.5432, 20.6683) -> (40.7861, 20.5957)
  line L607 (40.7861, 20.5957) -> (41.0283, 20.5108)
  line L608 (41.0283, 20.5108) -> (41.2698, 20.4147)
  line L609 (41.2698, 20.4147) -> (41.5104, 20.3084)
  line L610 (41.5104, 20.3084) -> (41.7502, 20.1925)
  line L611 (41.7502, 20.1925) -> (41.9889, 20.0674)
  line L612 (41.9889, 20.0674) -> (42.2264, 19.9336)
  line L613 (42.2264, 19.9336) -> (42.4038, 19.8276)
  line L614 (42.4038, 19.8276) -> (42.3616, 19.2919)
  line L615 (42.3616, 19.2919) -> (42.1699, 19.215)
  line L616 (42.1699, 19.215) -> (41.9143, 19.1199)
  line L617 (41.9143, 19.1199) -> (41.659, 19.0338)
  line L618 (41.659, 19.0338) -> (41.4041, 18.9568)
  line L619 (41.4041, 18.9568) -> (41.1497, 18.8894)
  line L620 (41.1497, 18.8894) -> (40.8962, 18.8323)
  line L621 (40.8962, 18.8323) -> (40.6437, 18.7863)
  line L622 (40.6437, 18.7863) -> (40.3924, 18.7526)
  line L623 (40.3924, 18.7526) -> (40.2674, 18.741)
  line L624 (40.2674, 18.741) -> (40.1429, 18.7335)
  line L625 (40.1429, 18.7335) -> (40.019, 18.7307)
  line L626 (40.019, 18.7307) -> (39.9573, 18.7315)
  line L627 (39.9573, 18.7315) -> (39.8959, 18.7343)
  line L628 (39.8959, 18.7343) -> (39.7957, 18.4624)
  line L629 (39.7957, 18.4624) -> (39.7404, 18.1135)
  line L630 (39.7404, 18.1135) -> (39.7517, 17.824)
  line L631 (39.7517, 17.824) -> (39.8109, 17.8076)
  line L632 (39.8109, 17.8076) -> (39.8699, 17.7894)
  line L633 (39.8699, 17.7894) -> (39.9869, 17.7484)
  line L634 (39.9869, 17.7484) -> (40.103, 17.7028)
  line L635 (40.103, 17.7028) -> (40.2183, 17.6531)
  line L636 (40.2183, 17.6531) -> (40.4468, 17.5434)
  line L637 (40.4468, 17.5434) -> (40.6728, 17.4216)
  line L638 (40.6728, 17.4216) -> (40.8963, 17.289)
  line L639 (40.8963, 17.289) -> (41.1173, 17.1463)
  line L640 (41.1173, 17.1463) -> (41.336, 16.9944)
  line L641 (41.336, 16.9944) -> (41.5521, 16.8335)
  line L642 (41.5521, 16.8335) -> (41.7658, 16.6641)
  line L643 (41.7658, 16.6641) -> (41.9244, 16.5317)
  line L644 (41.9244, 16.5317) -> (41.799, 16.0092)
  line L645 (41.799, 16.0092) -> (41.5976, 15.9632)
  line L646 (41.5976, 15.9632) -> (41.3303, 15.9093)
  line L647 (41.3303, 15.9093) -> (41.0646, 15.8641)
  line L648 (41.0646, 15.8641) -> (40.8008, 15.828)
  line L649 (40.8008, 15.828) -> (40.5391, 15.8012)
  line L650 (40.5391, 15.8012) -> (40.2797, 15.7845)
  line L651 (40.2797, 15.7845) -> (40.0231, 15.7786)
  line L652 (40.0231, 15.7786) -> (39.7697, 15.7846)
  line L653 (39.7697, 15.7846) -> (39.6444, 15.7927)
  line L654 (39.6444, 15.7927) -> (39.5202, 15.8047)
  line L655 (39.5202, 15.8047) -> (39.3974, 15.8214)
  line L656 (39.3974, 15.8214) -> (39.3366, 15.8318)
  line L657 (39.3366, 15.8318) -> (39.2764, 15.8442)
  line L658 (39.2764, 15.8442) -> (39.1349, 15.5913)
  line L659 (39.1349, 15.5913) -> (39.0257, 15.2554)
  line L660 (39.0257, 15.2554) -> (38.9916, 14.9676)
  line L661 (38.9916, 14.9676) -> (39.0476, 14.9422)
  line L662 (39.0476, 14.9422) -> (39.1029, 14.915)
  line L663 (39.1029, 14.915) -> (39.212, 14.8562)
  line L664 (39.212, 14.8562) -> (39.3196, 14.7929)
  line L665 (39.3196, 14.7929) -> (39.4257, 14.7259)
  line L666 (39.4257, 14.7259) -> (39.6343, 14.5818)
  line L667 (39.6343, 14.5818) -> (39.8384, 14.4261)
  line L668 (39.8384, 14.4261) -> (40.0384, 14.2601)
  line L669 (40.0384, 14.2601) -> (40.2344, 14.0847)
  line L670 (40.2344, 14.0847) -> (40.4266, 13.9004)
  line L671 (40.4266, 13.9004) -> (40.6149, 13.7077)
  line L672 (40.6149, 13.7077) -> (40.7995, 13.507)
  line L673 (40.7995, 13.507) -> (40.9354, 13.3514)
  line L674 (40.9354, 13.3514) -> (40.7298, 12.8549)
  line L675 (40.7298, 12.8549) -> (40.5236, 12.841)
  line L676 (40.5236, 12.841) -> (40.2512, 12.8296)
  line L677 (40.2512, 12.8296) -> (39.9817, 12.8265)
  line L678 (39.9817, 12.8265) -> (39.7155, 12.8321)
  line L679 (39.7155, 12.8321) -> (39.4528, 12.8466)
  line L680 (39.4528, 12.8466) -> (39.1941, 12.8707)
  line L681 (39.1941, 12.8707) -> (38.9397, 12.9049)
  line L682 (38.9397, 12.9049) -> (38.6903, 12.9505)
  line L683 (38.6903, 12.9505) -> (38.5678, 12.9781)
  line L684 (38.5678, 12.9781) -> (38.4471, 13.0095)
  line L685 (38.4471, 13.0095) -> (38.3284, 13.0451)
  line L686 (38.3284, 13.0451) -> (38.27, 13.0649)
  line L687 (38.27, 13.0649) -> (38.2124, 13.0865)
  line L688 (38.2124, 13.0865) -> (38.0331, 12.8589)
  line L689 (38.0331, 12.8589) -> (37.8727, 12.5442)
  line L690 (37.8727, 12.5442) -> (37.794, 12.2654)
  line L691 (37.794, 12.2654) -> (37.8453, 12.2315)
  line L692 (37.8453, 12.2315) -> (37.8957, 12.1959)
  line L693 (37.8957, 12.1959) -> (37.9943, 12.1208)
  line L694 (37.9943, 12.1208) -> (38.0906, 12.0415)
  line L695 (38.0906, 12.0415) -> (38.1849, 11.9586)
  line L696 (38.1849, 11.9586) -> (38.3684, 11.7837)
  line L697 (38.3684, 11.7837) -> (38.5456, 11.5981)
  line L698 (38.5456, 11.5981) -> (38.7172, 11.4028)
  line L699 (38.7172, 11.4028) -> (38.8834, 11.1989)
  line L700 (38.8834, 11.1989) -> (39.0443, 10.9868)
  line L701 (39.0443, 10.9868) -> (39.2002, 10.7669)
  line L702 (39.2002, 10.7669) -> (39.3511, 10.5398)
  line L703 (39.3511, 10.5398) -> (39.4611, 10.3649)
  line L704 (39.4611, 10.3649) -> (39.1803, 9.9067)
  line L705 (39.1803, 9.9067) -> (38.9745, 9.9252)
  line L706 (38.9745, 9.9252) -> (38.7037, 9.9566)
  line L707 (38.7037, 9.9566) -> (38.437, 9.9957)
  line L708 (38.437, 9.9957) -> (38.175, 10.0428)
  line L709 (38.175, 10.0428) -> (37.9178, 10.0983)
  line L710 (37.9178, 10.0983) -> (37.666, 10.1625)
  line L711 (37.666, 10.1625) -> (37.4201, 10.2362)
  line L712 (37.4201, 10.2362) -> (37.1809, 10.3202)
  line L713 (37.1809, 10.3202) -> (37.0642, 10.3666)
  line L714 (37.0642, 10.3666) -> (36.9499, 10.4164)
  line L715 (36.9499, 10.4164) -> (36.8382, 10.4702)
  line L716 (36.8382, 10.4702) -> (36.7836, 10.499)
  line L717 (36.7836, 10.499) -> (36.7301, 10.5293)
  line L718 (36.7301, 10.5293) -> (36.5174, 10.3326)
  line L719 (36.5174, 10.3326) -> (36.3098, 10.0468)
  line L720 (36.3098, 10.0468) -> (36.1884, 9.7837)
  line L721 (36.1884, 9.7837) -> (36.2338, 9.7422)
  line L722 (36.2338, 9.7422) -> (36.278, 9.6992)
  line L723 (36.278, 9.6992) -> (36.3636, 9.6096)
  line L724 (36.3636, 9.6096) -> (36.4464, 9.5162)
  line L725 (36.4464, 9.5162) -> (36.5266, 9.4196)
  line L726 (36.5266, 9.4196) -> (36.6804, 9.2181)
  line L727 (36.6804, 9.2181) -> (36.8264, 9.007)
  line L728 (36.8264, 9.007) -> (36.9653, 8.7874)
  line L729 (36.9653, 8.7874) -> (37.0975, 8.5599)
  line L730 (37.0975, 8.5599) -> (37.2234, 8.3252)
  line L731 (37.2234, 8.3252) -> (37.343, 8.0837)
  line L732 (37.343, 8.0837) -> (37.4565, 7.8358)
  line L733 (37.4565, 7.8358) -> (37.5377, 7.6459)
  line L734 (37.5377, 7.6459) -> (37.1887, 7.2372)
  line L735 (37.1887, 7.2372) -> (36.9883, 7.2877)
  line L736 (36.9883, 7.2877) -> (36.7257, 7.361)
  line L737 (36.7257, 7.361) -> (36.4685, 7.4414)
  line L738 (36.4685, 7.4414) -> (36.217, 7.5289)
  line L739 (36.217, 7.5289) -> (35.9717, 7.6239)
  line L740 (35.9717, 7.6239) -> (35.733, 7.7268)
  line L741 (35.733, 7.7268) -> (35.5016, 7.838)
  line L742 (35.5016, 7.838) -> (35.2786, 7.9584)
  line L743 (35.2786, 7.9584) -> (35.1706, 8.0225)
  line L744 (35.1706, 8.0225) -> (35.0654, 8.0896)
  line L745 (35.0654, 8.0896) -> (34.9635, 8.1602)
  line L746 (34.9635, 8.1602) -> (34.9141, 8.1971)
  line L747 (34.9141, 8.1971) -> (34.8661, 8.2354)
  line L748 (34.8661, 8.2354) -> (34.6252, 8.0744)
  line L749 (34.6252, 8.0744) -> (34.3754, 7.8246)
  line L750 (34.3754, 7.8246) -> (34.2144, 7.5837)
  line L751 (34.2144, 7.5837) -> (34.2527, 7.5357)
  line L752 (34.2527, 7.5357) -> (34.2896, 7.4863)
  line L753 (34.2896, 7.4863) -> (34.3602, 7.3844)
  line L754 (34.3602, 7.3844) -> (34.4273, 7.2792)
  line L755 (34.4273, 7.2792) -> (34.4914, 7.1712)
  line L756 (34.4914, 7.1712) -> (34.6118, 6.9482)
  line L757 (34.6118, 6.9482) -> (34.723, 6.7168)
  line L758 (34.723, 6.7168) -> (34.8259, 6.4781)
  line L759 (34.8259, 6.4781) -> (34.9209, 6.2328)
  line L760 (34.9209, 6.2328) -> (35.0084, 5.9813)
  line L761 (35.0084, 5.9813) -> (35.0888, 5.7241)
  line L762 (35.0888, 5.7241) -> (35.1621, 5.4615)
  line L763 (35.1621, 5.4615) -> (35.2126, 5.2611)
  line L764 (35.2126, 5.2611) -> (34.804, 4.9122)
  line L765 (34.804, 4.9122) -> (34.614, 4.9934)
  line L766 (34.614, 4.9934) -> (34.3661, 5.1069)
  line L767 (34.3661, 5.1069) -> (34.1246, 5.2265)
  line L768 (34.1246, 5.2265) -> (33.8899, 5.3523)
  line L769 (33.8899, 5.3523) -> (33.6624, 5.4845)
  line L770 (33.6624, 5.4845) -> (33.4428, 5.6234)
  line L771 (33.4428, 5.6234) -> (33.2317, 5.7694)
  line L772 (33.2317, 5.7694) -> (33.0302, 5.9233)
  line L773 (33.0302, 5.9233) -> (32.9336, 6.0035)
  line L774 (32.9336, 6.0035) -> (32.8402, 6.0862)
  line L775 (32.8402, 6.0862) -> (32.7506, 6.1718)
  line L776 (32.7506, 6.1718) -> (32.7076, 6.216)
  line L777 (32.7076, 6.216) -> (32.6661, 6.2614)
  line L778 (32.6661, 6.2614) -> (32.403, 6.14)
  line L779 (32.403, 6.14) -> (32.1173, 5.9324)
  line L780 (32.1173, 5.9324) -> (31.9205, 5.7197)
  line L781 (31.9205, 5.7197) -> (31.9509, 5.6662)
  line L782 (31.9509, 5.6662) -> (31.9796, 5.6116)
  line L783 (31.9796, 5.6116) -> (32.0334, 5.5)
  line L784 (32.0334, 5.5) -> (32.0832, 5.3856)
  line L785 (32.0832, 5.3856) -> (32.1296, 5.2689)
  line L786 (32.1296, 5.2689) -> (32.2137, 5.0298)
  line L787 (32.2137, 5.0298) -> (32.2873, 4.7839)
  line L788 (32.2873, 4.7839) -> (32.3515, 4.532)
  line L789 (32.3515, 4.532) -> (32.407, 4.2749)
  line L790 (32.407, 4.2749) -> (32.4541, 4.0128)
  line L791 (32.4541, 4.0128) -> (32.4932, 3.7462)
  line L792 (32.4932, 3.7462) -> (32.5246, 3.4753)
  line L793 (32.5246, 3.4753) -> (32.5431, 3.2695)
  line L794 (32.5431, 3.2695) -> (32.0849, 2.9888)
  line L795 (32.0849, 2.9888) -> (31.91, 3.0987)
  line L796 (31.91, 3.0987) -> (31.6829, 3.2496)
  line L797 (31.6829, 3.2496) -> (31.4631, 3.4055)
  line L798 (31.4631, 3.4055) -> (31.2509, 3.5664)
  line L799 (31.2509, 3.5664) -> (31.047, 3.7326)
  line L800 (31.047, 3.7326) -> (30.8518, 3.9042)
  line L801 (30.8518, 3.9042) -> (30.6661, 4.0814)
  line L802 (30.6661, 4.0814) -> (30.4912, 4.2649)
  line L803 (30.4912, 4.2649) -> (30.4083, 4.3592)
  line L804 (30.4083, 4.3592) -> (30.329, 4.4555)
  line L805 (30.329, 4.4555) -> (30.2539, 4.5541)
  line L806 (30.2539, 4.5541) -> (30.2183, 4.6045)
  line L807 (30.2183, 4.6045) -> (30.1845, 4.6558)
  line L808 (30.1845, 4.6558) -> (29.9056, 4.5771)
  line L809 (29.9056, 4.5771) -> (29.5909, 4.4167)
  line L810 (29.5909, 4.4167) -> (29.3633, 4.2374)
  line L811 (29.3633, 4.2374) -> (29.3849, 4.1799)
  line L812 (29.3849, 4.1799) -> (29.4047, 4.1215)
  line L813 (29.4047, 4.1215) -> (29.4404, 4.0027)
  line L814 (29.4404, 4.0027) -> (29.4717, 3.882)
  line L815 (29.4717, 3.882) -> (29.4993, 3.7595)
  line L816 (29.4993, 3.7595) -> (29.5449, 3.5101)
  line L817 (29.5449, 3.5101) -> (29.5791, 3.2557)
  line L818 (29.5791, 3.2557) -> (29.6032, 2.997)
  line L819 (29.6032, 2.997) -> (29.6178, 2.7343)
  line L820 (29.6178, 2.7343) -> (29.6233, 2.4681)
  line L821 (29.6233, 2.4681) -> (29.6202, 2.1986)
  line L822 (29.6202, 2.1986) -> (29.6088, 1.9262)
  line L823 (29.6088, 1.9262) -> (29.5949, 1.72)
  line L824 (29.5949, 1.72) -> (29.0984, 1.5144)
  line L825 (29.0984, 1.5144) -> (28.9428, 1.6503)
  line L826 (28.9428, 1.6503) -> (28.7421, 1.8349)
  line L827 (28.7421, 1.8349) -> (28.5494, 2.0233)
  line L828 (28.5494, 2.0233) -> (28.3651, 2.2154)
  line L829 (28.3651, 2.2154) -> (28.1897, 2.4115)
  line L830 (28.1897, 2.4115) -> (28.0237, 2.6115)
  line L831 (28.0237, 2.6115) -> (27.868, 2.8156)
  line L832 (27.868, 2.8156) -> (27.724, 3.0241)
  line L833 (27.724, 3.0241) -> (27.6569, 3.1303)
  line L834 (27.6569, 3.1303) -> (27.5936, 3.2378)
  line L835 (27.5936, 3.2378) -> (27.5349, 3.3469)
  line L836 (27.5349, 3.3469) -> (27.5076, 3.4023)
  line L837 (27.5076, 3.4023) -> (27.4822, 3.4583)
  line L838 (27.4822, 3.4583) -> (27.1944, 3.4241)
  line L839 (27.1944, 3.4241) -> (26.8585, 3.315)
  line L840 (26.8585, 3.315) -> (26.6057, 3.1734)
  line L841 (26.6057, 3.1734) -> (26.618, 3.1132)
  line L842 (26.618, 3.1132) -> (26.6284, 3.0524)
  line L843 (26.6284, 3.0524) -> (26.6451, 2.9296)
  line L844 (26.6451, 2.9296) -> (26.6571, 2.8054)
  line L845 (26.6571, 2.8054) -> (26.6652, 2.6801)
  line L846 (26.6652, 2.6801) -> (26.6713, 2.4267)
  line L847 (26.6713, 2.4267) -> (26.6653, 2.1701)
  line L848 (26.6653, 2.1701) -> (26.6486, 1.9107)
  line L849 (26.6486, 1.9107) -> (26.6219, 1.649)
  line L850 (26.6219, 1.649) -> (26.5857, 1.3852)
  line L851 (26.5857, 1.3852) -> (26.5405, 1.1195)
  line L852 (26.5405, 1.1195) -> (26.4866, 0.8522)
  line L853 (26.4866, 0.8522) -> (26.4406, 0.6508)
  line L854 (26.4406, 0.6508) -> (25.9181, 0.5254)
  line L855 (25.9181, 0.5254) -> (25.7857, 0.684)
  line L856 (25.7857, 0.684) -> (25.6163, 0.8977)
  line L857 (25.6163, 0.8977) -> (25.4555, 1.1139)
  line L858 (25.4555, 1.1139) -> (25.3035, 1.3325)
  line L859 (25.3035, 1.3325) -> (25.1608, 1.5536)
  line L860 (25.1608, 1.5536) -> (25.0282, 1.777)
  line L861 (25.0282, 1.777) -> (24.9064, 2.003)
  line L862 (24.9064, 2.003) -> (24.7967, 2.2315)
  line L863 (24.7967, 2.2315) -> (24.7471, 2.3469)
  line L864 (24.7471, 2.3469) -> (24.7014, 2.463)
  line L865 (24.7014, 2.463) -> (24.6605, 2.58)
  line L866 (24.6605, 2.58) -> (24.6422, 2.6389)
  line L867 (24.6422, 2.6389) -> (24.6258, 2.6981)
  line L868 (24.6258, 2.6981) -> (24.3363, 2.7094)
  line L869 (24.3363, 2.7094) -> (23.9874, 2.6542)
  line L870 (23.9874, 2.6542) -> (23.7155, 2.554)
  line L871 (23.7155, 2.554) -> (23.7183, 2.4925)
  line L872 (23.7183, 2.4925) -> (23.7191, 2.4309)
  line L873 (23.7191, 2.4309) -> (23.7163, 2.3069)
  line L874 (23.7163, 2.3069) -> (23.7088, 2.1824)
  line L875 (23.7088, 2.1824) -> (23.6972, 2.0574)
  line L876 (23.6972, 2.0574) -> (23.6635, 1.8061)
  line L877 (23.6635, 1.8061) -> (23.6175, 1.5536)
  line L878 (23.6175, 1.5536) -> (23.5604, 1.3001)
  line L879 (23.5604, 1.3001) -> (23.4931, 1.0457)
  line L880 (23.4931, 1.0457) -> (23.4161, 0.7908)
  line L881 (23.4161, 0.7908) -> (23.3299, 0.5355)
  line L882 (23.3299, 0.5355) -> (23.2348, 0.2799)
  line L883 (23.2348, 0.2799) -> (23.1579, 0.0882)
  line L884 (23.1579, 0.0882) -> (22.6222, 0.046)
  line L885 (22.6222, 0.046) -> (22.5162, 0.2234)
  line L886 (22.5162, 0.2234) -> (22.3824, 0.461)
  line L887 (22.3824, 0.461) -> (22.2573, 0.6996)
  line L888 (22.2573, 0.6996) -> (22.1414, 0.9394)
  line L889 (22.1414, 0.9394) -> (22.0351, 1.18)
  line L890 (22.0351, 1.18) -> (21.9391, 1.4215)
  line L891 (21.9391, 1.4215) -> (21.8541, 1.6637)
  line L892 (21.8541, 1.6637) -> (21.7815, 1.9066)
  line L893 (21.7815, 1.9066) -> (21.7505, 2.0283)
  line L894 (21.7505, 2.0283) -> (21.7236, 2.1501)
  line L895 (21.7236, 2.1501) -> (21.7014, 2.2721)
  line L896 (21.7014, 2.2721) -> (21.6926, 2.3331)
  line L897 (21.6926, 2.3331) -> (21.6857, 2.3942)
  line L898 (21.6857, 2.3942) -> (21.4015, 2.4506)
  line L899 (21.4015, 2.4506) -> (21.0483, 2.4506)
  line L900 (21.0483, 2.4506) -> (20.7641, 2.3942)
  line L901 (20.7641, 2.3942) -> (20.7572, 2.3331)
  line L902 (20.7572, 2.3331) -> (20.7484, 2.2721)
  line L903 (20.7484, 2.2721) -> (20.7262, 2.1501)
  line L904 (20.7262, 2.1501) -> (20.6993, 2.0283)
  line L905 (20.6993, 2.0283) -> (20.6683, 1.9066)
  line L906 (20.6683, 1.9066) -> (20.5957, 1.6637)
  line L907 (20.5957, 1.6637) -> (20.5108, 1.4215)
  line L908 (20.5108, 1.4215) -> (20.4147, 1.18)
  line L909 (20.4147, 1.18) -> (20.3084, 0.9394)
  line L910 (20.3084, 0.9394) -> (20.1925, 0.6996)
  line L911 (20.1925, 0.6996) -> (20.0674, 0.461)
  line L912 (20.0674, 0.461) -> (19.9336, 0.2234)
  line L913 (19.9336, 0.2234) -> (19.8276, 0.046)
  line L914 (19.8276, 0.046) -> (19.2919, 0.0882)
  line L915 (19.2919, 0.0882) -> (19.215, 0.2799)
  line L916 (19.215, 0.2799) -> (19.1199, 0.5355)
  line L917 (19.1199, 0.5355) -> (19.0338, 0.7908)
  line L918 (19.0338, 0.7908) -> (18.9568, 1.0457)
  line L919 (18.9568, 1.0457) -> (18.8894, 1.3001)
  line L920 (18.8894, 1.3001) -> (18.8323, 1.5536)
  line L921 (18.8323, 1.5536) -> (18.7863, 1.8061)
  line L922 (18.7863, 1.8061) -> (18.7526, 2.0574)
  line L923 (18.7526, 2.0574) -> (18.741, 2.1824)
  line L924 (18.741, 2.1824) -> (18.7335, 2.3069)
  line L925 (18.7335, 2.3069) -> (18.7307, 2.4309)
  line L926 (18.7307, 2.4309) -> (18.7315, 2.4925)
  line L927 (18.7315, 2.4925) -> (18.7343, 2.554)
  line L928 (18.7343, 2.554) -> (18.4624, 2.6542)
  line L929 (18.4624, 2.6542) -> (18.1135, 2.7094)
  line L930 (18.1135, 2.7094) -> (17.824, 2.6981)
  line L931 (17.824, 2.6981) -> (17.8076, 2.6389)
  line L932 (17.8076, 2.6389) -> (17.7894, 2.58)
  line L933 (17.7894, 2.58) -> (17.7484, 2.463)
  line L934 (17.7484, 2.463) -> (17.7028, 2.3469)
  line L935 (17.7028, 2.3469) -> (17.6531, 2.2315)
  line L936 (17.6531, 2.2315) -> (17.5434, 2.003)
  line L937 (17.5434, 2.003) -> (17.4216, 1.777)
  line L938 (17.4216, 1.777) -> (17.289, 1.5536)
  line L939 (17.289, 1.5536) -> (17.1463, 1.3325)
  line L940 (17.1463, 1.3325) -> (16.9944, 1.1139)
  line L941 (16.9944, 1.1139) -> (16.8335, 0.8977)
  line L942 (16.8335, 0.8977) -> (16.6641, 0.684)
  line L943 (16.6641, 0.684) -> (16.5317, 0.5254)
  line L944 (16.5317, 0.5254) -> (16.0092, 0.6508)
  line L945 (16.0092, 0.6508) -> (15.9632, 0.8522)
  line L946 (15.9632, 0.8522) -> (15.9093, 1.1195)
  line L947 (15.9093, 1.1195) -> (15.8641, 1.3852)
  line L948 (15.8641, 1.3852) -> (15.828, 1.649)
  line L949 (15.828, 1.649) -> (15.8012, 1.9107)
  line L950 (15.8012, 1.9107) -> (15.7845, 2.1701)
  line L951 (15.7845, 2.1701) -> (15.7786, 2.4267)
  line L952 (15.7786, 2.4267) -> (15.7846, 2.6801)
  line L953 (15.7846, 2.6801) -> (15.7927, 2.8054)
  line L954 (15.7927, 2.8054) -> (15.8047, 2.9296)